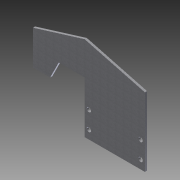
# Autodesk Inventor part: plate_metal_hook
Saved by Autodesk Inventor 2011 (Build 150239000, 239)
## iProperties
Created: 2013-01-17
Part Number: plate_metal_hook
Document SubType Name: Modeling
Designer: Christopher
Density: 1 g/cm^3
Author: Christopher
Autodesk Inventor part; units mm, degrees
ref_plane "YZ Plane" through (0, 0, 0) normal (1, 0, 0) x (0, 1, 0)
ref_plane "XZ Plane" through (0, 0, 0) normal (0, 1, 0) x (-1, 0, 0)
ref_plane "XY Plane" through (0, 0, 0) normal (0, 0, 1) x (1, 0, 0)
sketch "Sketch1" plane through (0, 0, 0) normal (0, 0, 1) x (1, 0, 0)
  line L0 (37.9991, 25.4) -> (37.9991, -50.8)
  line L1 (37.9991, -50.8) -> (126.8991, -50.8)
  line L2 (-12.8009, 0) -> (-38.2009, 0)
  line L3 (-38.2009, 0) -> (-38.2009, 50.8)
  line L4 (-12.8009, 0) -> (-0.1009, 25.4)
  line L5 (-0.1009, 25.4) -> (37.9991, 25.4)
  line L6 (37.9991, 74.2462) -> (126.8991, 50.8)
  line L7 (37.9991, 74.2462) -> (-38.2009, 50.8)
  line L8 (126.8991, 50.8) -> (126.8991, -50.8)
  point P0 (0, 0)
  point P1 (120.5491, -38.1)
  point P2 (120.5491, -12.7)
  point P3 (44.3491, -12.7)
  point P4 (44.3491, -38.1)
  dimension "d2" = 76.2
  dimension "d3" = 88.9
  dimension "d5" = 25.4
  dimension "d6" = 50.8
  dimension "d9" = 76.2
  dimension "d10" = 25.4
  dimension "d11" = 12.7
  dimension "d12" = 6.35
  constraints: 18 end point, 4 perpendicular, 3 horizontal alignment, 2 vertical alignment
  measures "d2" distance of L0.start L0.end
  measures "d3" distance of L0.end L1.end
  measures "d5" distance of L2.start L2.end
  measures "d6" distance of L2.end L3.end
  measures "d9" distance of point (120.549, -38.1) point (44.349, -38.1)
  measures "d10" distance of point (44.349, -38.1) point (44.349, -12.7)
  measures "d11" distance from line of L1 point (44.349, -38.1)
  measures "d12" distance from line of L0 point (44.349, -38.1)
extrude "Extrusion1" add sketch "Sketch1" against normal blind 3.175
hole "Hole1" at (120.5491, -38.1, 0) at (120.5491, -12.7, 0) at (44.3491, -12.7, 0) at (44.3491, -38.1, 0) direction (0, 0, -1) diameter 6.35 depth 25.4 tip angle 118
body "Solid1"
